Autodesk Inventor part; units mm, degrees
(part 2 of 2)
sketch "Sketch7" plane through (0, 0, 0) normal (0, 0, 1) x (1, 0, 0)
  line L0 (49.5999, 19) -> (79.846, 19) construction
  line L1 (79.846, 19) -> (79.846, 10.1748) construction
  line L2 (79.846, 10.1748) -> (49.5999, 10.1748) construction
  line L3 (49.5999, 10.1748) -> (49.5999, 19) construction
  line L4 (1, 0) -> (98.0599, 0) projected
  line L5 (101.5999, 3.81) -> (101.5999, 38.0999) projected
  line L6 (71.1843, 33.2803) -> (76.9638, 33.2803) construction
  line L7 (76.9638, 33.2803) -> (76.9638, 31.6428) construction
  line L8 (76.9638, 31.6428) -> (71.1843, 31.6428) construction
  line L9 (71.1843, 31.6428) -> (71.1843, 33.2803) construction
  line L10 (49.5946, 15.5) -> (50.9391, 19)
  line L11 (50.9391, 19) -> (51.4406, 19)
  line L12 (51.4406, 19) -> (52.8705, 15.5)
  line L13 (52.8705, 15.5) -> (52.3423, 15.5)
  line L14 (52.3423, 15.5) -> (51.9368, 16.5591)
  line L15 (51.9368, 16.5591) -> (50.4696, 16.5591)
  line L16 (50.4696, 16.5591) -> (50.0855, 15.5)
  line L17 (50.0855, 15.5) -> (49.5946, 15.5)
  line L18 (50.603, 16.9352) -> (51.7928, 16.9352)
  line L19 (51.7928, 16.9352) -> (51.4246, 17.9062)
  spline S0 degree 2 poles (51.4246, 17.9062) (51.2592, 18.3491) (51.1792, 18.6319) knots 0 0 0 1 1 1
  spline S1 degree 2 poles (51.1792, 18.6319) (51.1098, 18.2957) (50.9898, 17.9623) knots 0 0 0 1 1 1
  line L20 (50.9898, 17.9623) -> (50.603, 16.9352)
  line L21 (53.18, 15.5) -> (53.18, 18.037)
  line L22 (53.18, 18.037) -> (53.5668, 18.037)
  line L23 (53.5668, 18.037) -> (53.5668, 17.6528)
  spline S2 degree 2 poles (53.5668, 17.6528) (53.7135, 17.9223) (53.9643, 18.093) (54.1163, 18.093) knots 0 0 0 1 2 2 2
  spline S3 degree 2 poles (54.1163, 18.093) (54.3324, 18.093) (54.5565, 17.9569) knots 0 0 0 1 1 1
  line L24 (54.5565, 17.9569) -> (54.4071, 17.5568)
  spline S4 degree 2 poles (54.4071, 17.5568) (54.2497, 17.6502) (54.0923, 17.6502) knots 0 0 0 1 1 1
  spline S5 degree 2 poles (54.0923, 17.6502) (53.9509, 17.6502) (53.7295, 17.4794) (53.6815, 17.33) knots 0 0 0 1 2 2 2
  spline S6 degree 2 poles (53.6815, 17.33) (53.6095, 17.1006) (53.6095, 16.8285) knots 0 0 0 1 1 1
  line L25 (53.6095, 16.8285) -> (53.6095, 15.5)
  line L26 (53.6095, 15.5) -> (53.18, 15.5)
  line L27 (56.4585, 15.5) -> (56.4585, 15.8201)
  spline S7 degree 2 poles (56.4585, 15.8201) (56.2185, 15.444) (55.7489, 15.444) knots 0 0 0 1 1 1
  spline S8 degree 2 poles (55.7489, 15.444) (55.4448, 15.444) (54.938, 15.7774) (54.6579, 16.3777) (54.6579, 16.7671) knots 0 0 0 1 2 3 3 3
  spline S9 degree 2 poles (54.6579, 16.7671) (54.6579, 17.146) (54.9113, 17.7649) (55.4155, 18.093) (55.7276, 18.093) knots 0 0 0 1 2 3 3 3
  spline S10 degree 2 poles (55.7276, 18.093) (55.957, 18.093) (56.3145, 17.9009) (56.4265, 17.7462) knots 0 0 0 1 2 2 2
  line L28 (56.4265, 17.7462) -> (56.4265, 19)
  line L29 (56.4265, 19) -> (56.856, 19)
  line L30 (56.856, 19) -> (56.856, 15.5)
  line L31 (56.856, 15.5) -> (56.4585, 15.5)
  spline S11 degree 2 poles (55.1007, 16.7671) (55.1007, 16.279) (55.5115, 15.7961) (55.7916, 15.7961) knots 0 0 0 1 2 2 2
  spline S12 degree 2 poles (55.7916, 15.7961) (56.0717, 15.7961) (56.4665, 16.2576) (56.4665, 16.7298) knots 0 0 0 1 2 2 2
  spline S13 degree 2 poles (56.4665, 16.7298) (56.4665, 17.25) (56.0664, 17.7382) (55.7729, 17.7382) knots 0 0 0 1 2 2 2
  spline S14 degree 2 poles (55.7729, 17.7382) (55.4848, 17.7382) (55.1007, 17.2687) (55.1007, 16.7671) knots 0 0 0 1 2 2 2
  line L32 (59.1903, 15.5) -> (59.1903, 15.8735)
  spline S15 degree 2 poles (59.1903, 15.8735) (58.8941, 15.444) (58.3873, 15.444) knots 0 0 0 1 1 1
  spline S16 degree 2 poles (58.3873, 15.444) (58.1632, 15.444) (57.7737, 15.6147) (57.5843, 15.8761) (57.547, 16.0655) knots 0 0 0 1 2 3 3 3
  spline S17 degree 2 poles (57.547, 16.0655) (57.5203, 16.1909) (57.5203, 16.4657) knots 0 0 0 1 1 1
  line L33 (57.5203, 16.4657) -> (57.5203, 18.037)
  line L34 (57.5203, 18.037) -> (57.9498, 18.037)
  line L35 (57.9498, 18.037) -> (57.9498, 16.6311)
  spline S18 degree 2 poles (57.9498, 16.6311) (57.9498, 16.295) (57.9765, 16.1776) knots 0 0 0 1 1 1
  spline S19 degree 2 poles (57.9765, 16.1776) (58.0165, 16.0069) (58.2779, 15.8148) (58.4726, 15.8148) knots 0 0 0 1 2 2 2
  spline S20 degree 2 poles (58.4726, 15.8148) (58.6647, 15.8148) (59.0035, 16.0122) (59.1449, 16.3537) (59.1449, 16.6791) knots 0 0 0 1 2 3 3 3
  line L36 (59.1449, 16.6791) -> (59.1449, 18.037)
  line L37 (59.1449, 18.037) -> (59.5744, 18.037)
  line L38 (59.5744, 18.037) -> (59.5744, 15.5)
  line L39 (59.5744, 15.5) -> (59.1903, 15.5)
  line L40 (60.252, 15.5) -> (60.252, 18.037)
  line L41 (60.252, 18.037) -> (60.6815, 18.037)
  line L42 (60.6815, 18.037) -> (60.6815, 15.5)
  line L43 (60.6815, 15.5) -> (60.252, 15.5)
  line L44 (60.252, 18.5065) -> (60.252, 19)
  line L45 (60.252, 19) -> (60.6815, 19)
  line L46 (60.6815, 19) -> (60.6815, 18.5065)
  line L47 (60.6815, 18.5065) -> (60.252, 18.5065)
  line L48 (61.3351, 15.5) -> (61.3351, 18.037)
  line L49 (61.3351, 18.037) -> (61.7219, 18.037)
  line L50 (61.7219, 18.037) -> (61.7219, 17.6768)
  spline S21 degree 2 poles (61.7219, 17.6768) (62.002, 18.093) (62.5275, 18.093) knots 0 0 0 1 1 1
  spline S22 degree 2 poles (62.5275, 18.093) (62.7569, 18.093) (63.1411, 17.9276) (63.3332, 17.6608) (63.3705, 17.4768) knots 0 0 0 1 2 3 3 3
  spline S23 degree 2 poles (63.3705, 17.4768) (63.3945, 17.3567) (63.3945, 17.0579) knots 0 0 0 1 1 1
  line L51 (63.3945, 17.0579) -> (63.3945, 15.5)
  line L52 (63.3945, 15.5) -> (62.965, 15.5)
  line L53 (62.965, 15.5) -> (62.965, 17.0419)
  spline S24 degree 2 poles (62.965, 17.0419) (62.965, 17.3034) (62.8637, 17.5648) (62.6102, 17.7195) (62.4368, 17.7195) knots 0 0 0 1 2 3 3 3
  spline S25 degree 2 poles (62.4368, 17.7195) (62.1621, 17.7195) (61.7646, 17.37) (61.7646, 16.8845) knots 0 0 0 1 2 2 2
  line L54 (61.7646, 16.8845) -> (61.7646, 15.5)
  line L55 (61.7646, 15.5) -> (61.3351, 15.5)
  spline S26 degree 2 poles (63.8934, 16.7698) (63.8934, 17.4714) (64.2855, 17.8102) knots 0 0 0 1 1 1
  spline S27 degree 2 poles (64.2855, 17.8102) (64.611, 18.093) (65.0805, 18.093) knots 0 0 0 1 1 1
  spline S28 degree 2 poles (65.0805, 18.093) (65.6034, 18.093) (66.2676, 17.4074) (66.2676, 16.8045) knots 0 0 0 1 2 2 2
  spline S29 degree 2 poles (66.2676, 16.8045) (66.2676, 16.3163) (65.9742, 15.7534) (65.414, 15.444) (65.0805, 15.444) knots 0 0 0 1 2 3 3 3
  spline S30 degree 2 poles (65.0805, 15.444) (64.5496, 15.444) (63.8934, 16.1269) (63.8934, 16.7698) knots 0 0 0 1 2 2 2
  spline S31 degree 2 poles (64.3362, 16.7671) (64.3362, 16.2816) (64.7604, 15.7961) (65.0805, 15.7961) knots 0 0 0 1 2 2 2
  spline S32 degree 2 poles (65.0805, 15.7961) (65.4006, 15.7961) (65.8248, 16.2843) (65.8248, 16.7832) knots 0 0 0 1 2 2 2
  spline S33 degree 2 poles (65.8248, 16.7832) (65.8248, 17.2527) (65.3979, 17.7382) (65.0805, 17.7382) knots 0 0 0 1 2 2 2
  spline S34 degree 2 poles (65.0805, 17.7382) (64.7604, 17.7382) (64.3362, 17.2553) (64.3362, 16.7671) knots 0 0 0 1 2 2 2
  line L56 (49.9627, 9.992) -> (49.9627, 13.492)
  line L57 (49.9627, 13.492) -> (50.659, 13.492)
  line L58 (50.659, 13.492) -> (51.4887, 11.0138)
  spline S35 degree 2 poles (51.4887, 11.0138) (51.6034, 10.667) (51.6567, 10.4962) knots 0 0 0 1 1 1
  spline S36 degree 2 poles (51.6567, 10.4962) (51.7154, 10.6856) (51.8435, 11.0564) knots 0 0 0 1 1 1
  line L59 (51.8435, 11.0564) -> (52.6838, 13.492)
  line L60 (52.6838, 13.492) -> (53.3053, 13.492)
  line L61 (53.3053, 13.492) -> (53.3053, 9.992)
  line L62 (53.3053, 9.992) -> (52.8598, 9.992)
  line L63 (52.8598, 9.992) -> (52.8598, 12.9212)
  line L64 (52.8598, 12.9212) -> (51.8381, 9.992)
  line L65 (51.8381, 9.992) -> (51.422, 9.992)
  line L66 (51.422, 9.992) -> (50.4082, 12.9718)
  line L67 (50.4082, 12.9718) -> (50.4082, 9.992)
  line L68 (50.4082, 9.992) -> (49.9627, 9.992)
  line L69 (54.0603, 9.992) -> (54.0603, 13.492)
  line L70 (54.0603, 13.492) -> (56.5946, 13.492)
  line L71 (56.5946, 13.492) -> (56.5946, 13.0786)
  line L72 (56.5946, 13.0786) -> (54.5245, 13.0786)
  line L73 (54.5245, 13.0786) -> (54.5245, 12.0088)
  line L74 (54.5245, 12.0088) -> (56.4639, 12.0088)
  line L75 (56.4639, 12.0088) -> (56.4639, 11.5953)
  line L76 (56.4639, 11.5953) -> (54.5245, 11.5953)
  line L77 (54.5245, 11.5953) -> (54.5245, 10.4055)
  line L78 (54.5245, 10.4055) -> (56.6746, 10.4055)
  line L79 (56.6746, 10.4055) -> (56.6746, 9.992)
  line L80 (56.6746, 9.992) -> (54.0603, 9.992)
  line L81 (58.9528, 11.3632) -> (58.9528, 11.7767)
  line L82 (58.9528, 11.7767) -> (60.4334, 11.7767)
  line L83 (60.4334, 11.7767) -> (60.4334, 10.4802)
  spline S37 degree 2 poles (60.4334, 10.4802) (60.0919, 10.2081) (59.3663, 9.9334) (58.9848, 9.9334) knots 0 0 0 1 2 2 2
  spline S38 degree 2 poles (58.9848, 9.9334) (58.47, 9.9334) (57.627, 10.3762) (57.1975, 11.2112) (57.1975, 11.726) knots 0 0 0 1 2 3 3 3
  spline S39 degree 2 poles (57.1975, 11.726) (57.1975, 12.2382) (57.6243, 13.1239) (58.4273, 13.5534) (58.9502, 13.5534) knots 0 0 0 1 2 3 3 3
  spline S40 degree 2 poles (58.9502, 13.5534) (59.329, 13.5534) (59.9425, 13.308) (60.2893, 12.8678) (60.38, 12.513) knots 0 0 0 1 2 3 3 3
  line L84 (60.38, 12.513) -> (59.9639, 12.3983)
  spline S41 degree 2 poles (59.9639, 12.3983) (59.8838, 12.6651) (59.6518, 12.9718) (59.2169, 13.1559) (58.9528, 13.1559) knots 0 0 0 1 2 3 3 3
  spline S42 degree 2 poles (58.9528, 13.1559) (58.6354, 13.1559) (58.1712, 12.9638) (57.8884, 12.6464) (57.8084, 12.4596) knots 0 0 0 1 2 3 3 3
  spline S43 degree 2 poles (57.8084, 12.4596) (57.675, 12.1342) (57.675, 11.7554) knots 0 0 0 1 1 1
  spline S44 degree 2 poles (57.675, 11.7554) (57.675, 11.2885) (57.9978, 10.6563) (58.614, 10.3522) (58.9582, 10.3522) knots 0 0 0 1 2 3 3 3
  spline S45 degree 2 poles (58.9582, 10.3522) (59.2596, 10.3522) (59.8332, 10.5843) (59.9799, 10.715) knots 0 0 0 1 2 2 2
  line L85 (59.9799, 10.715) -> (59.9799, 11.3632)
  line L86 (59.9799, 11.3632) -> (58.9528, 11.3632)
  line L87 (60.7348, 9.992) -> (62.0794, 13.492)
  line L88 (62.0794, 13.492) -> (62.5809, 13.492)
  line L89 (62.5809, 13.492) -> (64.0108, 9.992)
  line L90 (64.0108, 9.992) -> (63.4826, 9.992)
  line L91 (63.4826, 9.992) -> (63.0771, 11.0511)
  line L92 (63.0771, 11.0511) -> (61.6098, 11.0511)
  line L93 (61.6098, 11.0511) -> (61.2257, 9.992)
  line L94 (61.2257, 9.992) -> (60.7348, 9.992)
  line L95 (61.7432, 11.4273) -> (62.933, 11.4273)
  line L96 (62.933, 11.4273) -> (62.5649, 12.3983)
  spline S46 degree 2 poles (62.5649, 12.3983) (62.3995, 12.8411) (62.3194, 13.1239) knots 0 0 0 1 1 1
  spline S47 degree 2 poles (62.3194, 13.1239) (62.2501, 12.7878) (62.13, 12.4543) knots 0 0 0 1 1 1
  line L97 (62.13, 12.4543) -> (61.7432, 11.4273)
  line L98 (67.8202, 10.4055) -> (67.8202, 9.992)
  line L99 (67.8202, 9.992) -> (65.5073, 9.992)
  spline S48 degree 2 poles (65.5073, 9.992) (65.502, 10.1468) (65.558, 10.2908) knots 0 0 0 1 1 1
  spline S49 degree 2 poles (65.558, 10.2908) (65.646, 10.5282) (66.0355, 10.9844) (66.4037, 11.2859) knots 0 0 0 1 2 2 2
  spline S50 degree 2 poles (66.4037, 11.2859) (66.9719, 11.7554) (67.372, 12.2996) (67.372, 12.545) knots 0 0 0 1 2 2 2
  spline S51 degree 2 poles (67.372, 12.545) (67.372, 12.8011) (67.0066, 13.1506) (66.7131, 13.1506) knots 0 0 0 1 2 2 2
  spline S52 degree 2 poles (66.7131, 13.1506) (66.4037, 13.1506) (66.0329, 12.7771) (66.0302, 12.449) knots 0 0 0 1 2 2 2
  line L100 (66.0302, 12.449) -> (65.5874, 12.4943)
  spline S53 degree 2 poles (65.5874, 12.4943) (65.6327, 12.9878) (66.2249, 13.5054) (66.7238, 13.5054) knots 0 0 0 1 2 2 2
  spline S54 degree 2 poles (66.7238, 13.5054) (67.228, 13.5054) (67.8149, 12.9478) (67.8149, 12.5343) knots 0 0 0 1 2 2 2
  spline S55 degree 2 poles (67.8149, 12.5343) (67.8149, 12.3236) (67.6441, 11.9181) (67.244, 11.4699) (66.7825, 11.0778) knots 0 0 0 1 2 3 3 3
  spline S56 degree 2 poles (66.7825, 11.0778) (66.3957, 10.755) (66.1769, 10.5229) (66.1049, 10.4055) knots 0 0 0 1 2 2 2
  line L101 (66.1049, 10.4055) -> (67.8202, 10.4055)
  line L102 (68.2817, 10.9097) -> (68.7326, 10.9471)
  spline S57 degree 2 poles (68.7326, 10.9471) (68.7832, 10.6163) (69.146, 10.2855) (69.4048, 10.2855) knots 0 0 0 1 2 2 2
  spline S58 degree 2 poles (69.4048, 10.2855) (69.7196, 10.2855) (70.1464, 10.755) (70.1464, 11.1418) knots 0 0 0 1 2 2 2
  spline S59 degree 2 poles (70.1464, 11.1418) (70.1464, 11.51) (69.7356, 11.9368) (69.3995, 11.9368) knots 0 0 0 1 2 2 2
  spline S60 degree 2 poles (69.3995, 11.9368) (69.1914, 11.9368) (68.8579, 11.7474) (68.7619, 11.5953) knots 0 0 0 1 2 2 2
  line L103 (68.7619, 11.5953) -> (68.3591, 11.6487)
  line L104 (68.3591, 11.6487) -> (68.6979, 13.4467)
  line L105 (68.6979, 13.4467) -> (70.4372, 13.4467)
  line L106 (70.4372, 13.4467) -> (70.4372, 13.0359)
  line L107 (70.4372, 13.0359) -> (69.042, 13.0359)
  line L108 (69.042, 13.0359) -> (68.8526, 12.0968)
  spline S61 degree 2 poles (68.8526, 12.0968) (69.1674, 12.3156) (69.5142, 12.3156) knots 0 0 0 1 1 1
  spline S62 degree 2 poles (69.5142, 12.3156) (69.973, 12.3156) (70.6026, 11.6807) (70.6026, 11.1818) knots 0 0 0 1 2 2 2
  spline S63 degree 2 poles (70.6026, 11.1818) (70.6026, 10.7043) (70.3252, 10.3575) knots 0 0 0 1 1 1
  spline S64 degree 2 poles (70.3252, 10.3575) (69.989, 9.9334) (69.4075, 9.9334) knots 0 0 0 1 1 1
  spline S65 degree 2 poles (69.4075, 9.9334) (68.93, 9.9334) (68.3244, 10.4669) (68.2817, 10.9097) knots 0 0 0 1 2 2 2
  line L109 (73.2329, 12.633) -> (72.8061, 12.5984)
  spline S66 degree 2 poles (72.8061, 12.5984) (72.7474, 12.8518) (72.6434, 12.9692) knots 0 0 0 1 1 1
  spline S67 degree 2 poles (72.6434, 12.9692) (72.4673, 13.1532) (72.2112, 13.1532) knots 0 0 0 1 1 1
  spline S68 degree 2 poles (72.2112, 13.1532) (72.0058, 13.1532) (71.8511, 13.0385) knots 0 0 0 1 1 1
  spline S69 degree 2 poles (71.8511, 13.0385) (71.6483, 12.8918) (71.4136, 12.3209) (71.4082, 11.7954) knots 0 0 0 1 2 2 2
  spline S70 degree 2 poles (71.4082, 11.7954) (71.563, 12.0328) (72.0138, 12.2622) (72.2592, 12.2622) knots 0 0 0 1 2 2 2
  spline S71 degree 2 poles (72.2592, 12.2622) (72.6887, 12.2622) (73.2943, 11.63) (73.2943, 11.1285) knots 0 0 0 1 2 2 2
  spline S72 degree 2 poles (73.2943, 11.1285) (73.2943, 10.8003) (73.0088, 10.2348) (72.5127, 9.9334) (72.1979, 9.9334) knots 0 0 0 1 2 3 3 3
  spline S73 degree 2 poles (72.1979, 9.9334) (71.659, 9.9334) (70.9814, 10.723) (70.9814, 11.63) knots 0 0 0 1 2 2 2
  spline S74 degree 2 poles (70.9814, 11.63) (70.9814, 12.6437) (71.3576, 13.1052) knots 0 0 0 1 1 1
  spline S75 degree 2 poles (71.3576, 13.1052) (71.683, 13.5054) (72.2379, 13.5054) knots 0 0 0 1 1 1
  spline S76 degree 2 poles (72.2379, 13.5054) (72.6514, 13.5054) (73.1796, 13.0412) (73.2329, 12.633) knots 0 0 0 1 2 2 2
  spline S77 degree 2 poles (71.4749, 11.1258) (71.4749, 10.9044) (71.6643, 10.4989) (72.0005, 10.2855) (72.1872, 10.2855) knots 0 0 0 1 2 3 3 3
  spline S78 degree 2 poles (72.1872, 10.2855) (72.462, 10.2855) (72.8515, 10.7257) (72.8515, 11.1018) knots 0 0 0 1 2 2 2
  spline S79 degree 2 poles (72.8515, 11.1018) (72.8515, 11.4646) (72.4673, 11.8834) (72.1712, 11.8834) knots 0 0 0 1 2 2 2
  spline S80 degree 2 poles (72.1712, 11.8834) (71.8804, 11.8834) (71.4749, 11.4646) (71.4749, 11.1258) knots 0 0 0 1 2 2 2
  spline S81 degree 2 poles (73.7185, 11.718) (73.7185, 12.3396) (73.9746, 13.0972) (74.4761, 13.5054) (74.8602, 13.5054) knots 0 0 0 1 2 3 3 3
  spline S82 degree 2 poles (74.8602, 13.5054) (75.1403, 13.5054) (75.5672, 13.2786) (75.8419, 12.8518) (75.9993, 12.2382) (75.9993, 11.718) knots 0 0 0 1 2 3 4 4 4
  spline S83 degree 2 poles (75.9993, 11.718) (75.9993, 11.1018) (75.7459, 10.3442) (75.2417, 9.9334) (74.8602, 9.9334) knots 0 0 0 1 2 3 3 3
  spline S84 degree 2 poles (74.8602, 9.9334) (74.3534, 9.9334) (74.0653, 10.2935) knots 0 0 0 1 1 1
  spline S85 degree 2 poles (74.0653, 10.2935) (73.7185, 10.7337) (73.7185, 11.718) knots 0 0 0 1 1 1
  spline S86 degree 2 poles (74.1613, 11.718) (74.1613, 10.8537) (74.5641, 10.2855) (74.8602, 10.2855) knots 0 0 0 1 2 2 2
  spline S87 degree 2 poles (74.8602, 10.2855) (75.1537, 10.2855) (75.5565, 10.8564) (75.5565, 11.718) knots 0 0 0 1 2 2 2
  spline S88 degree 2 poles (75.5565, 11.718) (75.5565, 12.5824) (75.1537, 13.1506) (74.8549, 13.1506) knots 0 0 0 1 2 2 2
  spline S89 degree 2 poles (74.8549, 13.1506) (74.5588, 13.1506) (74.3827, 12.8998) knots 0 0 0 1 1 1
  spline S90 degree 2 poles (74.3827, 12.8998) (74.1613, 12.5797) (74.1613, 11.718) knots 0 0 0 1 1 1
  line L110 (71.316, 32.0593) -> (71.316, 33.2593)
  line L111 (71.316, 33.2593) -> (71.8483, 33.2593)
  spline S91 degree 2 poles (71.8483, 33.2593) (72.0083, 33.2593) (72.1757, 33.1943) (72.2754, 33.0306) (72.2754, 32.9318) knots 0 0 0 1 2 3 3 3
  spline S92 degree 2 poles (72.2754, 32.9318) (72.2754, 32.8038) (72.1099, 32.6291) (71.9379, 32.6053) knots 0 0 0 1 2 2 2
  spline S93 degree 2 poles (71.9379, 32.6053) (72.0001, 32.5751) (72.033, 32.5459) knots 0 0 0 1 1 1
  spline S94 degree 2 poles (72.033, 32.5459) (72.1025, 32.4818) (72.1647, 32.3858) knots 0 0 0 1 1 1
  line L112 (72.1647, 32.3858) -> (72.3724, 32.0593)
  line L113 (72.3724, 32.0593) -> (72.1739, 32.0593)
  line L114 (72.1739, 32.0593) -> (72.0147, 32.309)
  spline S95 degree 2 poles (72.0147, 32.309) (71.9452, 32.4169) (71.8556, 32.5312) (71.7843, 32.5779) (71.7477, 32.587) knots 0 0 0 1 2 3 3 3
  spline S96 degree 2 poles (71.7477, 32.587) (71.7202, 32.5925) (71.6589, 32.5925) knots 0 0 0 1 1 1
  line L115 (71.6589, 32.5925) -> (71.4751, 32.5925)
  line L116 (71.4751, 32.5925) -> (71.4751, 32.0593)
  line L117 (71.4751, 32.0593) -> (71.316, 32.0593)
  line L118 (71.4751, 32.7297) -> (71.8163, 32.7297)
  spline S97 degree 2 poles (71.8163, 32.7297) (71.9251, 32.7297) (72.0477, 32.7745) (72.1117, 32.8742) (72.1117, 32.9318) knots 0 0 0 1 2 3 3 3
  spline S98 degree 2 poles (72.1117, 32.9318) (72.1117, 33.0169) (71.9882, 33.1267) (71.8547, 33.1267) knots 0 0 0 1 2 2 2
  line L119 (71.8547, 33.1267) -> (71.4751, 33.1267)
  line L120 (71.4751, 33.1267) -> (71.4751, 32.7297)
  line L121 (72.5279, 32.0593) -> (72.5279, 33.2593)
  line L122 (72.5279, 33.2593) -> (73.3968, 33.2593)
  line L123 (73.3968, 33.2593) -> (73.3968, 33.1175)
  line L124 (73.3968, 33.1175) -> (72.687, 33.1175)
  line L125 (72.687, 33.1175) -> (72.687, 32.7508)
  line L126 (72.687, 32.7508) -> (73.3519, 32.7508)
  line L127 (73.3519, 32.7508) -> (73.3519, 32.609)
  line L128 (73.3519, 32.609) -> (72.687, 32.609)
  line L129 (72.687, 32.609) -> (72.687, 32.2011)
  line L130 (72.687, 32.2011) -> (73.4242, 32.2011)
  line L131 (73.4242, 32.2011) -> (73.4242, 32.0593)
  line L132 (73.4242, 32.0593) -> (72.5279, 32.0593)
  line L133 (73.5888, 32.4453) -> (73.7388, 32.4581)
  spline S99 degree 2 poles (73.7388, 32.4581) (73.7498, 32.3675) (73.8275, 32.2523) (73.9913, 32.1809) (74.0937, 32.1809) knots 0 0 0 1 2 3 3 3
  spline S100 degree 2 poles (74.0937, 32.1809) (74.1843, 32.1809) (74.3242, 32.2349) (74.3919, 32.3291) (74.3919, 32.3849) knots 0 0 0 1 2 3 3 3
  spline S101 degree 2 poles (74.3919, 32.3849) (74.3919, 32.4416) (74.3269, 32.5258) (74.251, 32.5541) knots 0 0 0 1 2 2 2
  spline S102 degree 2 poles (74.251, 32.5541) (74.2025, 32.5733) (73.8705, 32.6529) (73.8038, 32.6886) knots 0 0 0 1 2 2 2
  spline S103 degree 2 poles (73.8038, 32.6886) (73.7178, 32.7334) (73.6336, 32.8669) (73.6336, 32.9492) knots 0 0 0 1 2 2 2
  spline S104 degree 2 poles (73.6336, 32.9492) (73.6336, 33.0407) (73.737, 33.198) (73.9355, 33.2803) (74.0571, 33.2803) knots 0 0 0 1 2 3 3 3
  spline S105 degree 2 poles (74.0571, 33.2803) (74.1907, 33.2803) (74.3946, 33.1943) (74.5053, 33.027) (74.5089, 32.9218) knots 0 0 0 1 2 3 3 3
  line L134 (74.5089, 32.9218) -> (74.3571, 32.9099)
  spline S106 degree 2 poles (74.3571, 32.9099) (74.3452, 33.0242) (74.2025, 33.1404) (74.0635, 33.1404) knots 0 0 0 1 2 2 2
  spline S107 degree 2 poles (74.0635, 33.1404) (73.919, 33.1404) (73.7864, 33.0343) (73.7864, 32.9602) knots 0 0 0 1 2 2 2
  spline S108 degree 2 poles (73.7864, 32.9602) (73.7864, 32.8953) (73.833, 32.8532) knots 0 0 0 1 1 1
  spline S109 degree 2 poles (73.833, 32.8532) (73.8797, 32.812) (74.2684, 32.7242) (74.3407, 32.6913) knots 0 0 0 1 2 2 2
  spline S110 degree 2 poles (74.3407, 32.6913) (74.4449, 32.6428) (74.5446, 32.4947) (74.5446, 32.3986) knots 0 0 0 1 2 2 2
  spline S111 degree 2 poles (74.5446, 32.3986) (74.5446, 32.3026) (74.4349, 32.1334) (74.2291, 32.0392) (74.101, 32.0392) knots 0 0 0 1 2 3 3 3
  spline S112 degree 2 poles (74.101, 32.0392) (73.9373, 32.0392) (73.7178, 32.1343) (73.5925, 32.3245) (73.5888, 32.4453) knots 0 0 0 1 2 3 3 3
  line L135 (74.765, 32.0593) -> (74.765, 33.2593)
  line L136 (74.765, 33.2593) -> (75.6339, 33.2593)
  line L137 (75.6339, 33.2593) -> (75.6339, 33.1175)
  line L138 (75.6339, 33.1175) -> (74.9242, 33.1175)
  line L139 (74.9242, 33.1175) -> (74.9242, 32.7508)
  line L140 (74.9242, 32.7508) -> (75.5891, 32.7508)
  line L141 (75.5891, 32.7508) -> (75.5891, 32.609)
  line L142 (75.5891, 32.609) -> (74.9242, 32.609)
  line L143 (74.9242, 32.609) -> (74.9242, 32.2011)
  line L144 (74.9242, 32.2011) -> (75.6614, 32.2011)
  line L145 (75.6614, 32.2011) -> (75.6614, 32.0593)
  line L146 (75.6614, 32.0593) -> (74.765, 32.0593)
  line L147 (76.1855, 32.0593) -> (76.1855, 33.1175)
  line L148 (76.1855, 33.1175) -> (75.7904, 33.1175)
  line L149 (75.7904, 33.1175) -> (75.7904, 33.2593)
  line L150 (75.7904, 33.2593) -> (76.7416, 33.2593)
  line L151 (76.7416, 33.2593) -> (76.7416, 33.1175)
  line L152 (76.7416, 33.1175) -> (76.3446, 33.1175)
  line L153 (76.3446, 33.1175) -> (76.3446, 32.0593)
  line L154 (76.3446, 32.0593) -> (76.1855, 32.0593)
  dimension "d113" = 19
  dimension "d114" = 52
  constraints: 4 other
  measures "d113" distance between parallel lines of L4 L0
  measures "d114" distance between parallel lines of L5 L3
extrude "Text" add sketch "Sketch7" along normal blind 0.1
ref_plane "Work Plane1" through (-6.34, 37.9499, 5.375) normal (-1, 0, 0) x (0, -1, 0)
sketch "Sketch8" plane through (-6.34, 37.9499, 5.375) normal (-1, 0, 0) x (0, -1, 0)
  line L0 (6.05, 5.375) -> (-6.05, 5.375)
  line L1 (-6.05, 5.375) -> (-6.05, -5.375)
  line L2 (6.05, -5.375) -> (6.05, 5.375)
  line L3 (-6.05, -5.375) -> (6.05, -5.375)
  line L4 (4, -4.075) -> (-4, -4.075)
  arc A0 (4, -4.075) -> (4.5, -3.575) centre (4, -3.575) ccw
  line L5 (4.5, -2.5) -> (4.5, -3.575)
  line L6 (4.5, 0.5) -> (4.5, -2.5)
  line L7 (4.5, 2.0922) -> (4.5, 0.5)
  line L8 (2.5086, 4.1664) -> (4.4414, 2.2336)
  line L9 (-2.3672, 4.225) -> (2.3672, 4.225)
  line L10 (-4.4414, 2.2336) -> (-2.5086, 4.1664)
  line L11 (-4.5, 0.5) -> (-4.5, 2.0922)
  line L12 (-4.5, -2.5) -> (-4.5, 0.5)
  line L13 (-4.5, -3.575) -> (-4.5, -2.5)
  arc A1 (-4.5, -3.575) -> (-4, -4.075) centre (-4, -3.575) ccw
  arc A2 (-4.4414, 2.2336) -> (-4.5, 2.0922) centre (-4.3, 2.0922) ccw
  arc A3 (-2.3672, 4.225) -> (-2.5086, 4.1664) centre (-2.3672, 4.025) ccw
  arc A4 (2.5086, 4.1664) -> (2.3672, 4.225) centre (2.3672, 4.025) ccw
  line L14 (2.8, 1.375) -> (-2.8, 1.375)
  line L15 (2.8, -1.775) -> (2.8, 1.375)
  line L16 (-2.8, -1.775) -> (2.8, -1.775)
  line L17 (-2.8, 1.375) -> (-2.8, -1.775)
  arc A5 (4.5, 2.0922) -> (4.4414, 2.2336) centre (4.3, 2.0922) ccw
  constraints: 36 end point, 12 point on circle, 10 vertical, 6 centre point, 6 horizontal, 38 other
extrude "Extrusion15" add sketch "Sketch8" against normal blind 16.3
sketch "Sketch9" plane through (9.96, 37.9499, 5.375) normal (1, 0, 0) x (0, 0, -1)
  line L0 (-5.375, 6.05) -> (5.375, 6.05) projected
  line L1 (-5.375, -6.05) -> (-5.375, 6.05) projected
  line L2 (5.375, -6.05) -> (-5.375, -6.05) projected
  line L3 (5.375, 6.05) -> (5.375, -6.05) projected
extrude "Extrusion16" add sketch "Sketch9" against normal blind 5
body "Solid1"
